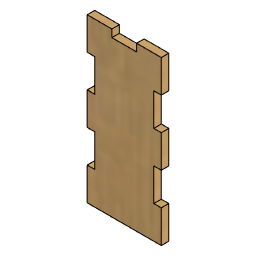
Balance Bot Assembled v16 (Autodesk Fusion 360 archive; units mm, degrees)
design "Panel B/D"
Autodesk Fusion 360 part; units mm, degrees
sketch "Sketch1" plane through (0, 0, 0) normal (0, 1, 0) x (1, 0, 0)
  line L0 (0, 0) -> (31.35, 0)
  line L1 (0, -68.89) -> (0, -55.1232)
  line L2 (0, -55.1232) -> (3.175, -55.1232)
  line L3 (3.175, -55.1232) -> (3.175, -41.3564)
  line L4 (3.175, -41.3564) -> (0, -41.3564)
  line L5 (0, -41.3564) -> (0, -27.5896)
  line L6 (0, -27.5896) -> (3.175, -27.5896)
  line L7 (3.175, -27.5896) -> (3.175, -13.8228)
  line L8 (3.175, -13.8228) -> (0, -13.8228)
  line L9 (0, -68.89) -> (0, -55.1232)
  line L10 (0, -41.3564) -> (0, -27.5896)
  line L11 (0, -13.8228) -> (0, 0)
  line L12 (31.35, -68.89) -> (31.35, -55.1232)
  line L13 (31.35, -55.1232) -> (28.175, -55.1232)
  line L14 (28.175, -55.1232) -> (28.175, -41.3564)
  line L15 (28.175, -41.3564) -> (31.35, -41.3564)
  line L16 (31.35, -41.3564) -> (31.35, -27.5896)
  line L17 (31.35, -27.5896) -> (28.175, -27.5896)
  line L18 (28.175, -27.5896) -> (28.175, -13.8228)
  line L19 (28.175, -13.8228) -> (31.35, -13.8228)
  line L20 (31.35, -13.8228) -> (31.35, 0)
  line L21 (31.35, -55.1232) -> (31.35, -68.89)
  line L22 (31.35, 0) -> (31.35, -13.8228)
  line L23 (31.35, -27.5896) -> (31.35, -41.3564)
  line L24 (0, -68.89) -> (10.4479, -68.89)
  line L25 (10.4479, -68.89) -> (10.4479, -65.715)
  line L26 (10.4479, -65.715) -> (20.8873, -65.715)
  line L27 (20.8873, -65.715) -> (20.8873, -68.89)
  line L28 (31.35, -68.89) -> (20.8873, -68.89)
  line L29 (10.4479, -68.89) -> (0, -68.89)
  dimension "d1" = 31.35
  dimension "d2" = 68.89
  dimension "d3" = 13.7668
  dimension "d4" = 3.175
  dimension "d5" = 13.7668
  dimension "d6" = 13.7668
  dimension "d7" = 13.7668
  dimension "d10" = 10.4479
  dimension "d11" = 3.175
  dimension "d12" = 10.4394
  constraint horizontal L0
  constraint vertical L22
  constraint horizontal L28
  constraint vertical L9
  constraint coincident L0.start L11.end
  constraint perpendicular L1 L28
  constraint perpendicular L2 L9
  constraint perpendicular L2 L3
  constraint coincident L4.end L9
  constraint perpendicular L4 L9
  constraint perpendicular L4 L5
  constraint perpendicular L3 L6
  constraint perpendicular L6 L7
  constraint coincident L8.end L9
  constraint perpendicular L8 L9
  constraint collinear L9 L10
  constraint collinear L10 L11
  constraint collinear L21 L22
  constraint collinear L22 L23
  constraint perpendicular L21 L24
  constraint perpendicular L24 L25
  constraint perpendicular L25 L26
  constraint perpendicular L27 L28
  constraint collinear L28 L29
  measures "d1" distance of L0.start L0.end
  measures "d2" distance of L0.start L1.start
  measures "d3" distance of L1.start L1.end
  measures "d4" distance of L1.end L2.end
  measures "d5" distance of L2.end L3.end
  measures "d6" distance of L4.end L5.end
  measures "d7" distance of L6.end L7.end
  measures "d10" distance of L1.start L24.end
  measures "d11" distance of L24.end L25.end
  measures "d12" distance of L25.end L26.end
extrude "Extrude1" add sketch "Sketch1" along normal blind 3.175
equation "d1 = 0.25 in + 25 mm"
equation "d2 = 0.25 in + 6 cm + 0.1 in"
equation "d10 = 1.234 in / 3"

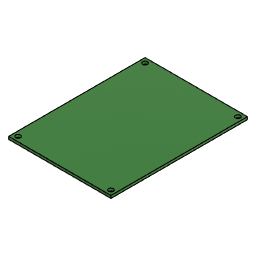
design "ProtoBoard"
Autodesk Fusion 360 part; units mm, degrees
sketch "Sketch1" plane through (0, 0, 0) normal (0, 0, 1) x (1, 0, 0)
  line L0 (0, 0) -> (60, 0)
  line L1 (60, 0) -> (60, 80)
  line L2 (60, 80) -> (0, 80)
  line L3 (0, 80) -> (0, 0)
  dimension "d1" = 60
  dimension "d2" = 80
  constraint horizontal L0
  constraint vertical L1
  constraint horizontal L2
  constraint vertical L3
  constraint coincident L0.start L3.end
  measures "d1" distance of L0.start L0.end
  measures "d2" distance of L0.start L2.end
extrude "Extrude1" add sketch "Sketch1" along normal blind 1.5
sketch "Sketch2" plane through (0, 0, 1.5) normal (0, 0, 1) x (-1, 0, 0)
  line L0 (0, -80) -> (0, 0)
  line L1 (0, 0) -> (-60, 0)
  line L2 (-60, 0) -> (-60, -80)
  line L3 (-60, -80) -> (0, -80)
  line L4 (0, -80) -> (-2.8, -80)
  line L5 (-2.8, -80) -> (-2.8, -77.2)
  line L6 (-2.8, -77.2) -> (0, -77.2)
  line L7 (0, -77.2) -> (0, -80)
  circle A0 centre (-2.8, -77.2) radius 1.4
  line L8 (-30, -80) -> (-30, 0)
  line L9 (-60, -40) -> (0, -40)
  circle A1 centre (-57.2, -77.2) radius 1.4
  circle A2 centre (-57.2, -2.8) radius 1.4
  circle A3 centre (-2.8, -2.8) radius 1.4
  dimension "d5" = 2.8
  dimension "d6" = 2.8
  dimension "d7" = 2.8
  constraint horizontal L4
  constraint vertical L5
  constraint horizontal L6
  constraint vertical L7
  constraint coincident L0.start L3.end
  constraint coincident L5.end L6.start
  constraint midpoint L3 L8.start
  constraint midpoint L1 L8.end
  constraint midpoint L2 L9.start
  constraint midpoint L0 L9.end
  constraint symmetric A0 L8 A1
  constraint symmetric A0 L9 A3
  constraint symmetric L9 A1 A2
  measures "d5" distance of L0.start L4.end
  measures "d6" distance of L0.start L6.end
  measures "d7" diameter of A0
extrude "Extrude2" cut sketch "Sketch2" against normal blind 2 contours L5 L6 A0 | L5 L6 A0 | A1 | A2 | A3

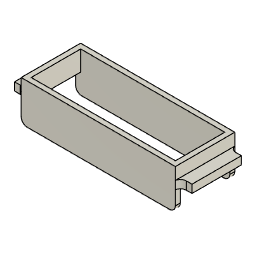
design "Coupler"
Autodesk Fusion 360 part; units mm, degrees
sketch "Sketch1" plane through (0, 0, 0) normal (0, 0, 1) x (1, 0, 0)
  line L0 (0, 0) -> (91.44, 0)
  line L1 (91.44, 0) -> (91.44, 31.3436)
  line L2 (91.44, 31.3436) -> (0, 31.3436)
  line L3 (0, 31.3436) -> (0, 0)
  line L4 (-3.175, -3.175) -> (94.615, -3.175)
  line L5 (94.615, -3.175) -> (94.615, 34.5186)
  line L6 (94.615, 34.5186) -> (-3.175, 34.5186)
  line L7 (-3.175, 34.5186) -> (-3.175, -3.175)
  dimension "d1" = 91.44
  dimension "d2" = 31.3436
  dimension "d3" = 3.175
  constraint horizontal L0
  constraint vertical L1
  constraint horizontal L2
  constraint vertical L3
  constraint coincident L0.start L3.end
  measures "d1" distance of L0.start L0.end
  measures "d2" distance of L0.start L2.end
extrude "Extrude1" add sketch "Sketch1" against normal blind 12.7
sketch "Sketch2" plane through (0, 0, -12.7) normal (0, 0, -1) x (1, 0, 0)
  line L0 (0, -31.3436) -> (0, 0)
  line L1 (0, 0) -> (91.44, 0)
  line L2 (91.44, 0) -> (91.44, -31.3436)
  line L3 (91.44, -31.3436) -> (0, -31.3436)
  line L4 (-3.175, 3.175) -> (-3.175, -34.5186)
  line L5 (-3.175, -34.5186) -> (94.615, -34.5186)
  line L6 (94.615, -34.5186) -> (94.615, 3.175)
  line L7 (94.615, 3.175) -> (-3.175, 3.175)
  line L8 (0, 0) -> (-3.175, 0)
  line L9 (0, -31.3436) -> (-3.175, -31.3436)
  line L10 (91.44, 0) -> (94.615, 0)
  line L11 (91.44, -31.3436) -> (94.615, -31.3436)
  constraint coincident L0.end L1.start
  constraint coincident L4 L8.end
  constraint perpendicular L4 L8
  constraint coincident L0.start L3.end
  constraint coincident L4 L9.end
  constraint perpendicular L4 L9
  constraint coincident L1.end L2.start
  constraint coincident L6 L10.end
  constraint perpendicular L6 L10
  constraint coincident L2.end L3.start
  constraint coincident L6 L11.end
  constraint perpendicular L6 L11
sketch "Sketch3" plane through (-3.175, 0, 0) normal (-1, 0, 0) x (0, -1, 0)
  line L0 (3.175, 0) -> (-34.5186, 0)
  line L1 (-34.5186, 0) -> (-34.5186, -12.7)
  line L2 (-34.5186, -12.7) -> (3.175, -12.7)
  line L3 (3.175, -12.7) -> (3.175, 0)
  line L4 (-34.5186, -12.7) -> (-31.3436, -12.7)
  line L5 (-31.3436, -12.7) -> (0.027, -12.7)
  line L6 (0.027, -12.7) -> (0.027, -7.62)
  line L7 (0.027, -7.62) -> (-31.3436, -7.62)
  line L8 (-31.3436, -7.62) -> (-31.3436, -12.7)
  dimension "d6" = 31.3706
  dimension "d7" = 5.08
  constraint coincident L1.end L2.start
  constraint coincident L2 L4.end
  constraint perpendicular L1 L4
  constraint horizontal L5
  constraint vertical L6
  constraint horizontal L7
  constraint vertical L8
  measures "d6" distance of L4.end L5.end
  measures "d7" distance of L4.end L7.end
extrude "Extrude2" add sketch "Sketch3" along normal blind 10.4902 contours L2 L5 L6 L7 L8
fillet "Fillet1" radius 3.81 2 edges at (-3.175, -0.027, -10.16) (-3.175, 31.3436, -10.16)
sketch "Sketch4" plane through (94.615, 0, 0) normal (1, 0, 0) x (0, 1, 0)
  line L0 (34.5186, 0) -> (-3.175, 0)
  line L1 (-3.175, 0) -> (-3.175, -12.7)
  line L2 (-3.175, -12.7) -> (34.5186, -12.7)
  line L3 (34.5186, -12.7) -> (34.5186, 0)
  line L4 (-3.175, -12.7) -> (0, -12.7)
  line L5 (0, -12.7) -> (31.3436, -12.7)
  line L6 (31.3436, -12.7) -> (31.3436, -7.62)
  line L7 (31.3436, -7.62) -> (0, -7.62)
  line L8 (0, -7.62) -> (0, -12.7)
  dimension "d12" = 31.3436
  dimension "d13" = 5.08
  constraint coincident L1.end L2.start
  constraint coincident L2 L4.end
  constraint perpendicular L1 L4
  constraint horizontal L5
  constraint vertical L6
  constraint horizontal L7
  constraint vertical L8
  measures "d12" distance of L4.end L5.end
  measures "d13" distance of L4.end L7.end
extrude "Extrude3" add sketch "Sketch4" along normal blind 10.4902 contours L2 L5 L6 L7 L8
fillet "Fillet2" radius 3.81 2 edges at (94.615, 0, -10.16) (94.615, 31.3436, -10.16)
extrude "Extrude4" add sketch "Sketch2" along normal blind 12.7 contours L3 L4 L5 L6 L9 L11 | L1 L4 L6 L7 L8 L10
fillet "Fillet3" radius 3.81 4 edges at (94.615, 32.9311, -25.4) (94.615, -1.5875, -25.4) (-3.175, 32.9311, -25.4) (-3.175, -1.5875, -25.4)
extrude "Extrude5" cut 1 faces at (105.1052, 20.8957, -11.0067) along direction (-1, 0, 0) blind 3.1496
extrude "Extrude6" cut 1 faces at (-13.6652, 10.4299, -9.3133) along direction (1, 0, 0) blind 3.1496

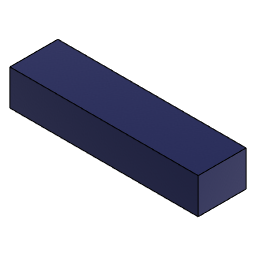
design "GN3 550 90c/180c LiPo approx."
Autodesk Fusion 360 part; units mm, degrees
sketch "Sketch1" plane through (0, 0, 0) normal (0, 0, 1) x (1, 0, 0)
  line L0 (0, 0) -> (69.85, 0)
  line L1 (69.85, 0) -> (69.85, 17.78)
  line L2 (69.85, 17.78) -> (0, 17.78)
  line L3 (0, 17.78) -> (0, 0)
  dimension "d1" = 69.85
  dimension "d2" = 17.78
  constraint horizontal L0
  constraint vertical L1
  constraint horizontal L2
  constraint vertical L3
  constraint coincident L0.start L3.end
  measures "d1" distance of L0.start L0.end
  measures "d2" distance of L0.start L2.end
extrude "Extrude1" add sketch "Sketch1" along normal blind 13.208

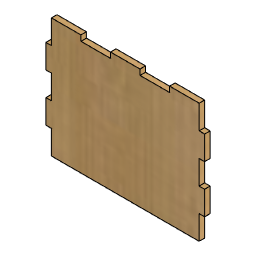
design "Panel A/C"
Autodesk Fusion 360 part; units mm, degrees
sketch "Sketch1" plane through (0, 0, 0) normal (0, 1, 0) x (1, 0, 0)
  line L0 (3.175, 0) -> (88.255, 0)
  line L1 (0, -55.0774) -> (3.175, -55.0774)
  line L2 (0, -41.3106) -> (3.175, -41.3106)
  line L3 (0, -27.5438) -> (3.175, -27.5438)
  line L4 (0, -13.777) -> (3.175, -13.777)
  line L5 (0, -55.0774) -> (0, -41.3106)
  line L6 (0, -27.5438) -> (0, -13.777)
  line L7 (3.175, 0) -> (3.175, -13.777)
  line L8 (3.175, -27.5438) -> (3.175, -41.3106)
  line L9 (3.175, -55.0774) -> (3.175, -68.89)
  line L10 (88.255, -55.0774) -> (88.255, -68.89)
  line L11 (91.43, -55.0774) -> (88.255, -55.0774)
  line L12 (91.43, -55.0774) -> (91.43, -41.3106)
  line L13 (91.43, -41.3106) -> (88.255, -41.3106)
  line L14 (88.255, -27.5438) -> (88.255, -41.3106)
  line L15 (91.43, -27.5438) -> (88.255, -27.5438)
  line L16 (91.43, -27.5438) -> (91.43, -13.777)
  line L17 (91.43, -13.777) -> (88.255, -13.777)
  line L18 (88.255, 0) -> (88.255, -13.777)
  line L19 (88.255, -55.0774) -> (88.255, -68.89)
  line L20 (88.255, 0) -> (88.255, -13.777)
  line L21 (88.255, -27.5438) -> (88.255, -41.3106)
  line L22 (3.175, -68.89) -> (20.183, -68.89)
  line L23 (20.183, -68.89) -> (20.183, -65.715)
  line L24 (20.183, -65.715) -> (37.201, -65.715)
  line L25 (37.201, -65.715) -> (37.201, -68.89)
  line L26 (37.201, -68.89) -> (54.219, -68.89)
  line L27 (54.219, -68.89) -> (54.219, -65.715)
  line L28 (54.219, -65.715) -> (71.237, -65.715)
  line L29 (71.237, -65.715) -> (71.237, -68.89)
  line L30 (20.183, -68.89) -> (3.175, -68.89)
  line L31 (88.255, -68.89) -> (71.237, -68.89)
  line L32 (54.219, -68.89) -> (37.201, -68.89)
  line L33 (3.175, -68.89) -> (20.193, -68.89)
  dimension "d1" = 88.255
  dimension "d3" = 3.175
  dimension "d4" = 13.777
  dimension "d5" = 13.7668
  dimension "d6" = 13.7668
  dimension "d7" = 13.7668
  dimension "d11" = 3.175
  dimension "d12" = 17.018
  dimension "d13" = 17.018
  dimension "d14" = 3.175
  dimension "d15" = 17.018
  dimension "d16" = 3.175
  dimension "d17" = 3.175
  dimension "d18" = 17.018
  dimension "d19" = 17.018
  constraint horizontal L0
  constraint vertical L20
  constraint horizontal L31
  constraint vertical L5
  constraint perpendicular L7 L31
  constraint coincident L1.end L7
  constraint perpendicular L1 L7
  constraint coincident L2.end L7
  constraint perpendicular L2 L7
  constraint coincident L3.start L5
  constraint coincident L3.end L7
  constraint perpendicular L3 L7
  constraint coincident L4.start L5
  constraint perpendicular L4 L7
  constraint collinear L5 L6
  constraint collinear L7 L8
  constraint collinear L8 L9
  constraint collinear L19 L20
  constraint collinear L20 L21
  constraint perpendicular L10 L22
  constraint perpendicular L22 L23
  constraint perpendicular L23 L24
  constraint perpendicular L25 L31
  constraint perpendicular L25 L26
  constraint perpendicular L27 L31
  constraint perpendicular L27 L28
  constraint perpendicular L29 L31
  constraint collinear L30 L31
  constraint collinear L31 L32
  constraint perpendicular L19 L33
  measures "d1" distance of origin L0.end
  measures "d3" distance of origin L0.start
  measures "d4" distance of origin L4.start
  measures "d5" distance of L3 L4.start
  measures "d6" distance of L2 L3.start
  measures "d7" distance of L1.start L2.start
  measures "d11" distance of L22.end L23.end
  measures "d12" distance of L23.end L24.end
  measures "d13" distance of L25.end L26.end
  measures "d14" distance of L26.end L27.end
  measures "d15" distance of L27.end L28.end
  measures "d16" distance of L16.end L17.end
  measures "d17" distance of L12.end L13.end
  measures "d18" distance of L9.end L33.end
  measures "d19" distance of L10.end L29.end
extrude "Extrude1" add sketch "Sketch1" along normal blind 3.175
equation "d1 = 0.2 in + 0.25 in + 80 mm - 0.125 in"
equation "d4 = 2.712 in / 5"
equation "d18 = 3.350 in / 5"

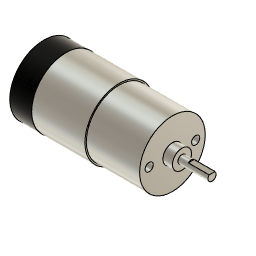
design "Motor Approx."
Autodesk Fusion 360 part; units mm, degrees
sketch "Sketch1" plane through (0, 0, 0) normal (1, 0, 0) x (0, 1, 0)
  circle A0 centre (0, 0) radius 12.5
  dimension "d1" = 25
  constraint coincident A0.centre origin
  measures "d1" diameter of A0
extrude "Extrude1" add sketch "Sketch1" along normal blind 19.5 makes body 1
sketch "Sketch2" plane through (19.5, 0, 0) normal (1, 0, 0) x (0, 1, 0)
  circle A0 centre (0, 0) radius 12.5
  circle A1 centre (0, 0) radius 12
  dimension "d4" = 24
  constraint coincident A0.centre A1.centre
  measures "d4" diameter of A1
extrude "Extrude2" add sketch "Sketch2" along normal blind 19.5 contours A1 bodies 1
sketch "Sketch3" plane through (39, 0, 0) normal (1, 0, 0) x (0, 1, 0)
  circle A0 centre (0, 0) radius 12
  circle A1 centre (0, 0) radius 3.5
  dimension "d7" = 7
  constraint coincident A0.centre A1.centre
  measures "d7" diameter of A1
extrude "Extrude3" add sketch "Sketch3" along normal blind 3.5 contours A1 bodies 1
sketch "Sketch4" plane through (42.5, 0, 0) normal (1, 0, 0) x (0, 1, 0)
  circle A0 centre (0, 0) radius 3.5
  circle A1 centre (0, 0) radius 1.5
  dimension "d10" = 3
  constraint coincident A0.centre A1.centre
  measures "d10" diameter of A1
extrude "Extrude4" add sketch "Sketch4" along normal blind 11 contours A1 bodies 1
sketch "Sketch5" plane through (53.5, 0, 0) normal (1, 0, 0) x (0, 1, 0)
  circle A0 centre (0, 0) radius 1.5
  line L0 (0, 0) -> (0, -1.5)
  line L1 (0, 0) -> (0, 1.5)
  line L2 (0, 1.5) -> (0, 1.05)
  line L3 (0, 1.05) -> (1.0712, 1.05)
  line L4 (0, 1.05) -> (-1.0712, 1.05)
  dimension "d13" = 1.5
  dimension "d14" = 0.45
  constraint coincident A0.centre L0.start
  constraint coincident A0 L0.end
  constraint vertical L0
  constraint parallel L0 L1
  constraint parallel L1 L2
  constraint coincident A0 L3.end
  constraint perpendicular L2 L3
  constraint coincident A0 L4.end
  constraint perpendicular L1 L4
  measures "d13" distance of A0.centre L1.end
  measures "d14" distance of L1.end L2.end
extrude "Extrude5" cut sketch "Sketch5" against normal blind 7.62 contours A0 L1 L2 L3 | A0 L1 L2 L4 bodies 1
extrude "Extrude6" add 1 faces at (0, -3.3879, -0.621) along direction (-1, 0, 0) blind 8 separate body on bodies 1 makes body 2
sketch "Sketch6" plane through (39, 0, 0) normal (1, 0, 0) x (0, 1, 0)
  circle A0 centre (0, 0) radius 3.5
  circle A1 centre (0, 0) radius 12
  line L0 (0, 0) -> (8.5, 0)
  line L1 (0, 0) -> (-8.5, 0)
  circle A2 centre (-8.5, 0) radius 1.5
  circle A3 centre (8.5, 0) radius 1.5
  dimension "d19" = 8.5
  dimension "d20" = 8.5
  dimension "d21" = 3
  dimension "d22" = 3
  constraint coincident A0.centre A1.centre
  constraint horizontal L0
  constraint parallel L0 L1
  constraint coincident L1.end A2.centre
  constraint coincident L0.end A3.centre
  measures "d19" distance of A0.centre L0.end
  measures "d20" distance of A0.centre L1.end
  measures "d21" diameter of A2
  measures "d22" diameter of A3
extrude "Extrude7" cut sketch "Sketch6" against normal blind 2.54 contours A2 | A3 bodies 1
equation "d8 = 7 mm / 2"
equation "d13 = 3 mm / 2"
equation "d19 = 17 mm / 2"
equation "d20 = 17 mm / 2"

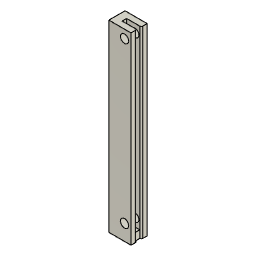
design "ProtoBoard Mount"
Autodesk Fusion 360 part; units mm, degrees
sketch "Sketch3" plane through (0, 0, 0) normal (0, 0, 1) x (1, 0, 0)
  line L0 (-40, -0.75) -> (-40, 0.75)
  line L1 (-40, -0.75) -> (-35.5, -0.75)
  line L2 (-35, -1.25) -> (-35, -2.25)
  line L3 (-35.5, -2.75) -> (-40, -2.75)
  line L4 (-40, -2.75) -> (-40, -0.75)
  line L5 (-40, 0.75) -> (-35.5, 0.75)
  line L6 (-35, 1.25) -> (-35, 2.25)
  line L7 (-35.5, 2.75) -> (-40, 2.75)
  line L8 (-40, 2.75) -> (-40, 0.75)
  line L9 (-40, 2.75) -> (-42.54, 2.75)
  line L10 (-42.54, 2.75) -> (-42.54, -2.75)
  line L11 (-42.54, -2.75) -> (-40, -2.75)
  line L12 (-40, -2.75) -> (-40, 2.75)
  line L13 (-35.5, -0.75) -> (-40, -0.75)
  line L14 (0, 0) -> (0, -3)
  line L15 (-35.5, -2.75) -> (-38.5, -2.75)
  line L16 (-35, -1.25) -> (-35, -2.25)
  arc A0 (-35, -1.25) -> (-35.5, -0.75) centre (-35.5, -1.25) ccw
  line L17 (-38.5, -0.75) -> (-35.5, -0.75)
  line L18 (-38.5, 0.75) -> (-35.5, 0.75)
  arc A1 (-35.5, 0.75) -> (-35, 1.25) centre (-35.5, 1.25) ccw
  line L19 (-35, 1.25) -> (-35, 2.25)
  line L20 (-35.5, 2.75) -> (-38.5, 2.75)
  line L21 (-35, 2.25) -> (-35, 2.75)
  line L22 (-35, 2.75) -> (-35.5, 2.75)
  line L23 (-35.5, -2.75) -> (-35, -2.75)
  line L24 (-35, -2.75) -> (-35, -2.25)
  line L25 (40, -2.75) -> (40, 2.75)
  line L26 (38.5, 0.75) -> (35.5, 0.75)
  line L27 (40, -2.75) -> (40, -0.75)
  line L28 (38.5, -0.75) -> (35.5, -0.75)
  line L29 (40, 0.75) -> (35.5, 0.75)
  line L30 (42.54, -2.75) -> (40, -2.75)
  line L31 (35, -1.25) -> (35, -2.25)
  line L32 (35.5, -2.75) -> (35, -2.75)
  line L33 (35, 1.25) -> (35, 2.25)
  line L34 (35.5, 2.75) -> (40, 2.75)
  line L35 (40, 2.75) -> (40, 0.75)
  line L36 (35, -2.75) -> (35, -2.25)
  line L37 (35.5, -2.75) -> (40, -2.75)
  line L38 (42.54, 2.75) -> (42.54, -2.75)
  line L39 (35, 1.25) -> (35, 2.25)
  line L40 (40, 2.75) -> (42.54, 2.75)
  line L41 (35, 2.25) -> (35, 2.75)
  line L42 (35, 2.75) -> (35.5, 2.75)
  line L43 (35.5, -0.75) -> (40, -0.75)
  arc A2 (35.5, -0.75) -> (35, -1.25) centre (35.5, -1.25) ccw
  line L44 (40, -0.75) -> (35.5, -0.75)
  line L45 (35.5, -2.75) -> (38.5, -2.75)
  line L46 (35, -1.25) -> (35, -2.25)
  arc A3 (35, 1.25) -> (35.5, 0.75) centre (35.5, 1.25) ccw
  line L47 (40, -0.75) -> (40, 0.75)
  line L48 (35.5, 2.75) -> (38.5, 2.75)
  dimension "d24" = 2
  dimension "d26" = 2
  dimension "d32" = 2.54
  dimension "d46" = 5
  dimension "d49" = 5
  dimension "d50" = 1.5
  dimension "d51" = 40
  constraint coincident L14.start origin
  constraint horizontal L1
  constraint vertical L2
  constraint horizontal L3
  constraint vertical L4
  constraint horizontal L5
  constraint vertical L6
  constraint horizontal L7
  constraint vertical L8
  constraint horizontal L9
  constraint vertical L10
  constraint horizontal L11
  constraint vertical L12
  constraint vertical L14
  constraint perpendicular L20 L21
  constraint perpendicular L21 L22
  constraint perpendicular L2 L23
  constraint perpendicular L23 L24
  constraint symmetric L0.end L14 L29.start
  constraint symmetric L0.start L14 L27.end
  constraint symmetric L3.end L14 L25.start
  constraint symmetric L7.end L14 L25.end
  constraint symmetric L9.end L14 L38.start
  constraint symmetric L10.end L14 L30.start
  constraint symmetric L14 L3.start L32.start
  constraint symmetric L14 L15.end L45.end
  constraint symmetric L14 L2.end L31.end
  constraint symmetric L14 L2.start L31.start
  constraint symmetric L14 L1.end L28.end
  constraint symmetric L14 A0 A2
  constraint symmetric L14 L17.start L28.start
  constraint symmetric L14 L18.start L26.start
  constraint symmetric L14 L5.end L26.end
  constraint symmetric L14 L6.start L33.start
  constraint symmetric L14 A1 A3
  constraint symmetric L14 L6.end L33.end
  constraint symmetric L14 L7.start L34.start
  constraint symmetric L14 L20.end L48.end
  constraint symmetric L14 L21.end L41.end
  constraint symmetric L14 L23.end L32.end
  measures "d24" distance of L0.start L3.end
  measures "d26" distance of L0.end L7.end
  measures "d32" distance of L7.end L9.end
  measures "d46" distance of L2 L12
  measures "d49" distance of L8 L19
  measures "d50" distance of L17 L18
  measures "d51" distance of L14.start L0
extrude "Extrude2" add sketch "Sketch3" along normal blind 60 contours L0 L4 L8 L9 L10 L11 L12 | L1 L2 L3 L4 L12 L13 L15 L16 A0 L17 L23 L24 | L5 L6 L7 L8 L12 L18 A1 L19 L20 L21 L22
sketch "Sketch5" plane through (0, 2.75, 0) normal (0, 1, 0) x (-1, 0, 0)
  line L0 (35, 0) -> (42.54, 0)
  line L1 (42.54, 0) -> (42.54, 60)
  line L2 (42.54, 60) -> (35, 60)
  line L3 (35, 60) -> (35, 0)
  line L4 (42.54, 0) -> (40, 0)
  line L5 (40, 0) -> (37.2, 0)
  line L6 (37.2, 0) -> (37.2, 2.8)
  circle A0 centre (37.2, 2.8) radius 1.4
  line L7 (0, 0) -> (0, 10)
  line L8 (42.54, 30) -> (27.8434, 30)
  circle A1 centre (-37.2, 2.8) radius 1.4
  circle A2 centre (37.2, 57.2) radius 1.4
  circle A3 centre (-37.2, 57.2) radius 1.4
  dimension "d52" = 2.8
  dimension "d53" = 2.8
  constraint coincident L0.end L1.start
  constraint coincident L0 L4.end
  constraint perpendicular L1 L4
  constraint perpendicular L1 L5
  constraint perpendicular L5 L6
  constraint coincident L6.end A0.centre
  constraint coincident L7.start origin
  constraint vertical L7
  constraint midpoint L1 L8.start
  constraint perpendicular L3 L8
  constraint symmetric A0 L7 A1
  constraint symmetric A0 L8 A2
  constraint symmetric L8 A1 A3
  measures "d52" distance of L4.end L5.end
  measures "d53" distance of L5.end L6.end
extrude "Extrude4" cut sketch "Sketch5" against normal blind 9 contours A0 | A2
extrude "Extrude5" add 1 faces at (-41.6933, 0.25, 0) along direction (0, 0, -1) blind 2.54
sketch "Sketch6" plane through (-40, 0, 0) normal (1, 0, 0) x (0, 1, 0)
  line L0 (0.75, -2.54) -> (0.75, 60)
  line L1 (0.75, 60) -> (-0.75, 60)
  line L2 (-0.75, 60) -> (-0.75, -2.54)
  line L3 (-0.75, -2.54) -> (0.75, -2.54)
  line L4 (0.75, -2.54) -> (-0.75, -2.54)
  line L5 (-0.75, -2.54) -> (-0.75, 0)
  line L6 (-0.75, 0) -> (0.75, 0)
  line L7 (0.75, 0) -> (0.75, -2.54)
  constraint horizontal L4
  constraint vertical L5
  constraint horizontal L6
  constraint vertical L7
  constraint coincident L2 L5.end
  constraint coincident L0.start L3.end
extrude "Extrude6" add sketch "Sketch6" along normal blind 4.5 contours L0 L2 L3 L4 L5 L6 L7

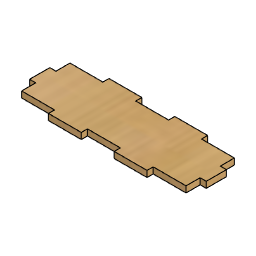
design "Lid"
Autodesk Fusion 360 part; units mm, degrees
sketch "Sketch2" plane through (0, 0, 0) normal (0, 0, 1) x (1, 0, 0)
  line L0 (91.44, 10.4479) -> (91.44, 20.8957)
  line L1 (0, 20.8957) -> (0, 10.4479)
  line L2 (3.175, 28.1686) -> (20.193, 28.1686)
  line L3 (37.211, 28.1686) -> (54.229, 28.1686)
  line L4 (20.193, 28.1686) -> (20.193, 31.3436)
  line L5 (37.211, 28.1686) -> (37.211, 31.3436)
  line L6 (54.229, 28.1686) -> (54.229, 31.3436)
  line L7 (71.247, 28.1686) -> (71.247, 31.3436)
  line L8 (3.175, 28.1686) -> (3.175, 20.8957)
  line L9 (3.175, 3.175) -> (3.175, 10.4479)
  line L10 (3.175, 10.4479) -> (0, 10.4479)
  line L11 (3.175, 20.8957) -> (0, 20.8957)
  line L12 (88.265, 3.175) -> (88.265, 10.4479)
  line L13 (88.265, 28.1686) -> (88.265, 20.8957)
  line L14 (88.265, 20.8957) -> (91.44, 20.8957)
  line L15 (88.265, 10.4479) -> (91.44, 10.4479)
  line L16 (20.193, 0) -> (37.211, 0)
  line L17 (54.229, 0) -> (71.247, 0)
  line L18 (71.247, 31.3436) -> (54.229, 31.3436)
  line L19 (37.211, 31.3436) -> (20.193, 31.3436)
  line L20 (3.175, 28.1686) -> (3.175, 20.8957)
  line L21 (3.175, 10.4479) -> (3.175, 3.175)
  line L22 (20.193, 3.175) -> (20.193, 0)
  line L23 (3.175, 3.175) -> (20.193, 3.175)
  line L24 (37.211, 3.175) -> (37.211, 0)
  line L25 (54.229, 3.175) -> (54.229, 0)
  line L26 (37.211, 3.175) -> (54.229, 3.175)
  line L27 (71.247, 3.175) -> (88.265, 3.175)
  line L28 (71.247, 3.175) -> (71.247, 0)
  line L29 (88.265, 3.175) -> (88.265, 10.4479)
  line L30 (88.265, 20.8957) -> (88.265, 28.1686)
  line L31 (88.265, 28.1686) -> (71.247, 28.1686)
  line L32 (54.229, 28.1686) -> (37.211, 28.1686)
  line L33 (20.193, 28.1686) -> (3.175, 28.1686)
  dimension "d21" = 85.09
  dimension "d22" = 24.9936
  dimension "d23" = 17.018
  dimension "d24" = 17.018
  dimension "d25" = 17.018
  dimension "d26" = 17.018
  constraint horizontal L16
  constraint vertical L0
  constraint horizontal L18
  constraint vertical L1
  constraint horizontal L31
  constraint perpendicular L20 L31
  constraint parallel L23 L31
  constraint parallel L20 L29
  constraint perpendicular L2 L29
  constraint perpendicular L3 L29
  constraint coincident L4.end L18
  constraint perpendicular L4 L18
  constraint coincident L5.end L18
  constraint perpendicular L5 L18
  constraint perpendicular L6 L18
  constraint perpendicular L7 L18
  constraint perpendicular L8 L16
  constraint perpendicular L9 L18
  constraint perpendicular L1 L10
  constraint perpendicular L1 L11
  constraint perpendicular L12 L18
  constraint perpendicular L13 L16
  constraint perpendicular L0 L14
  constraint perpendicular L0 L15
  constraint coincident L17.start L16
  constraint coincident L17.end L16
  constraint collinear L16 L17
  constraint collinear L18 L19
  constraint collinear L20 L21
  constraint collinear L23 L26
  constraint collinear L26 L27
  constraint collinear L29 L30
  constraint collinear L31 L32
  constraint collinear L32 L33
  measures "d21" distance of L9.start L12.start
  measures "d22" distance of L2.start L9.start
  measures "d23" distance of L2.start L2.end
  measures "d24" distance of L2.end L3.start
  measures "d25" distance of L3.start L3.end
  measures "d26" distance of L3.end L7.start
extrude "Extrude2" add sketch "Sketch2" along normal blind 3.175
extrude "Extrude1" [rolled back] along distance 3.175 taper angle 0
equation "d21 = 3.600 in - 0.25 in"
equation "d22 = 1.234 in - 0.25 in"
equation "d23 = 3.350 in / 5"
equation "d24 = 2.680 in / 4"
equation "d25 = 2.010 in / 3"
equation "d26 = 1.340 in / 2"

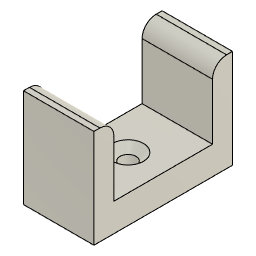
design "Battery Cradle"
Autodesk Fusion 360 part; units mm, degrees
sketch "Sketch1" plane through (0, 0, 0) normal (0, 0, 1) x (1, 0, 0)
  line L0 (0, 0) -> (12.7, 0)
  line L1 (12.7, 0) -> (12.7, 17.78)
  line L2 (12.7, 17.78) -> (0, 17.78)
  line L3 (0, 17.78) -> (0, 0)
  line L4 (0, 17.78) -> (12.7, 17.78)
  line L5 (12.7, 17.78) -> (12.7, 21.3868)
  line L6 (12.7, 21.3868) -> (0, 21.3868)
  line L7 (0, 21.3868) -> (0, 17.78)
  line L8 (0, 0) -> (12.7, 0)
  line L9 (12.7, 0) -> (12.7, -3.6068)
  line L10 (12.7, -3.6068) -> (0, -3.6068)
  line L11 (0, -3.6068) -> (0, 0)
  dimension "d1" = 12.7
  dimension "d2" = 17.78
  dimension "d11" = 3.6068
  dimension "d12" = 3.6068
  dimension "d13" = 24.9936
  constraint horizontal L0
  constraint vertical L1
  constraint horizontal L2
  constraint vertical L3
  constraint coincident L0.start L3.end
  constraint horizontal L4
  constraint vertical L5
  constraint horizontal L6
  constraint vertical L7
  constraint horizontal L8
  constraint vertical L9
  constraint horizontal L10
  constraint vertical L11
  measures "d1" distance of L0.start L0.end
  measures "d2" distance of L0.start L2.end
  measures "d11" distance of L2.end L6.end
  measures "d12" distance of L0.start L10.end
  measures "d13" distance of L6 L10
extrude "Extrude1" add sketch "Sketch1" along normal blind 5.08
extrude "Extrude2" add sketch "Sketch1" along normal blind 12.7 contours L0 L8 L9 L10 L11 | L2 L4 L5 L6 L7
extrude "Extrude3" add 2 faces at (4.2333, -1.2023, 12.7) (4.2333, 20.1845, 12.7) along direction (0, 0, 1) blind 5.08
sketch "Sketch2" plane through (0, 0, 17.78) normal (0, 0, 1) x (-1, 0, 0)
  line L0 (0, -21.3868) -> (0, -17.78)
  line L1 (0, -17.78) -> (-12.7, -17.78)
  line L2 (-12.7, -17.78) -> (-12.7, -21.3868)
  line L3 (-12.7, -21.3868) -> (0, -21.3868)
  line L4 (-6.35, -21.3868) -> (-6.35, -17.78)
  constraint midpoint L3 L4.start
  constraint midpoint L1 L4.end
fillet "Fillet1" radius 2.54 2 edges at (6.35, 0, 17.78) (6.35, 17.78, 17.78)
sketch "Sketch3" plane through (0, 0, 5.08) normal (0, 0, 1) x (-1, 0, 0)
  line L0 (-12.7, -17.78) -> (0, -17.78)
  line L1 (0, -17.78) -> (0, 0)
  line L2 (0, 0) -> (-12.7, 0)
  line L3 (-12.7, 0) -> (-12.7, -17.78)
  line L4 (0, 0) -> (-12.7, -17.78)
  line L5 (-12.7, 0) -> (0, -17.78)
  circle A0 centre (-6.35, -8.89) radius 1.45
  dimension "d16" = 2.9
  constraint coincident L1.end L2.start
  constraint coincident L0.start L3.end
  constraint coincident L2.end L3.start
  constraint coincident L0.end L1.start
  constraint midpoint L5 A0.centre
  measures "d16" diameter of A0
extrude "Extrude4" cut sketch "Sketch3" against normal blind 8.89 contours L4 L5 A0 | L4 L5 A0 | L4 L5 A0 | L4 L5 A0
chamfer "Chamfer1" distance 1.3462 angle 45 1 edges at (7.7019, 8.3657, 5.08)
